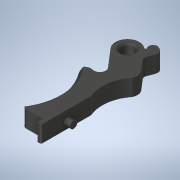
# Autodesk Inventor part: Trigger
Saved by Autodesk Inventor 2020.1 (Build 241239000, 239)
## iProperties
Created: 2019-07-16
Part Number: Trigger
Material: Generic
Document SubType Name: Modeling
Designer: Petar
Density: 1 g/cm^3
Appearance: Black Only
Mass: 1.77104 g
Surface Area: 13.1807 cm^2
Volume: 1.77104 cm^3
Author: Petar
Autodesk Inventor part; units mm, degrees
ref_plane "YZ Plane" through (0, 0, 0) normal (1, 0, 0) x (0, 1, 0)
ref_plane "XZ Plane" through (0, 0, 0) normal (0, 1, 0) x (-1, 0, 0)
sketch "Sketch1" plane through (0, 0, 0) normal (0, 1, 0) x (-1, 0, 0)
  arc A0 (0.6231, 32.7963) -> (2.0842, 14.5566) centre (15.636, 24.8205) ccw
  line L0 (-0.7016, 35) -> (-5.7016, 35)
  arc A1 (0.6231, 32.7963) -> (-0.7016, 35) centre (-0.7016, 33.5) ccw
  arc A2 (1.4227, 12.2493) -> (2.0842, 14.5566) centre (0.8884, 13.6509) ccw
  arc A3 (-9.0865, 8.0552) -> (-7.7016, 20) centre (-18.71, 15.2236) ccw
  line L1 (-7.7016, 37) -> (-7.7016, 20)
  arc A4 (-2.5532, -3.0792) -> (3.0381, 2.6019) centre (0, 0) ccw
  circle A5 centre (0, 0) radius 2.2
  arc A6 (-0.4832, 12.1334) -> (-2.3197, 8.8578) centre (-0.8007, 10.1588) ccw
  line L2 (3.0381, 2.6019) -> (-2.3197, 8.8578)
  line L3 (-5.8467, 0.6774) -> (-8.9592, 4.3116)
  arc A7 (-9.0865, 8.0552) -> (-8.9592, 4.3116) centre (-6.6806, 6.263) ccw
  line L4 (0, 0) -> (0, -31) construction
  line L5 (1.4227, 12.2493) -> (0.7686, 12)
  line L6 (-0.4832, 12.1334) -> (0.5112, 11.9735)
  arc A8 (0.5112, 11.9735) -> (0.7686, 12) centre (0.5905, 12.4672) ccw
  line L7 (3.7362, -42.8746) -> (-104.2638, 7.1254) construction
  line L8 (-104.2638, 7.1254) -> (-40.257, 145.38) construction
  line L9 (-40.257, 145.38) -> (67.743, 95.38) construction
  line L10 (67.743, 95.38) -> (3.7362, -42.8746) construction
  line L11 (-3.3359, -3.2768) -> (-4.3901, -5.8859) construction
  line L12 (-4.3901, -5.8859) -> (-7.1716, -4.7621)
  line L13 (-7.1716, -4.7621) -> (-5.5952, -0.8602)
  arc A9 (-5.5952, -0.8602) -> (-5.8467, 0.6774) centre (-6.986, -0.2983) ccw
  arc A10 (-2.5532, -3.0792) -> (-3.3359, -3.2768) centre (-2.8723, -3.4641) ccw
  line L14 (-7.7016, 37) -> (-6.2016, 37)
  line L15 (-6.2016, 37) -> (-6.2016, 35.5)
  arc A11 (-6.2016, 35.5) -> (-5.7016, 35) centre (-5.7016, 35.5) ccw
  arc A12 (-4.3901, -5.8859) -> (-3.3359, -3.2768) centre (-4.345, -4.3866) ccw
  point P0 (-7.7016, 35)
  point P1 (-3.0552, -2.5819)
  point P2 (-6.2016, 35)
  dimension "d5" = 7
  dimension "d6" = 15
  dimension "d7" = 8
  dimension "d8" = 4.4
  dimension "d9" = 2
  dimension "d10" = 35
  dimension "d14" = 3
  dimension "d18" = 12
  dimension "d93" = 3
  dimension "d94" = 1.5
  dimension "d96" = 22
  dimension "d109" = 0.5
  dimension "d115" = 0.7
  dimension "d116" = 150
  dimension "d121" = 0.5
  dimension "d123" = 1.5
  dimension "d124" = 2
  dimension "d140" = 1.5
  constraints: 25 point on circle, 24 end point, 18 tangent, 13 centre point, 5 point on line, 4 perpendicular, 3 coincident, 1 parallel, 1 vertical, 9 other
  measures "d5" distance of L0.start point (-7.702, 35)
  measures "d6" distance of point (-7.702, 35) L1.end
  measures "d7" diameter of A4
  measures "d8" diameter of A5
  measures "d9" radius of A6
  measures "d10" distance from line of L0 A4.centre
  measures "d14" radius of A7
  measures "d18" radius of A3
  measures "d93" distance between parallel lines of L13 L11
  measures "d94" radius of A9
  measures "d96" angle of L4 L11
  measures "d109" radius of A10
  measures "d115" distance of L5.start L5.end
  measures "d116" angle of L6 L5
  measures "d121" radius of A11
  measures "d123" distance of L1.start L14.end
  measures "d124" distance between parallel lines of L14 L0
  measures "d140" radius of A12
extrude "Extrusion1" add sketch "Sketch1" along normal mid plane 5.6
ref_plane "Work Plane1" through (-15.636, 0, 24.8205) normal (0, 0, -1) x (0, 1, 0)
sketch "Sketch2" plane through (-15.636, 0, 24.8205) normal (0, 0, -1) x (0, 1, 0)
  line L0 (-25.04, 0) -> (8.14, 0) construction
  line L1 (0, 15.636) -> (0, 0) construction
  line L2 (-19.6, 0) -> (3.3, 18.4018)
  line L3 (3.3, 18.4018) -> (3.3, 0)
  line L4 (2.8, 17) -> (2.8, 15.0129) construction
  line L5 (2.8, 17) -> (2.8, 18)
  line L6 (-2.8, 21.3376) -> (-2.8, 16.3376) construction
  line L7 (0, 15.75) -> (2.8, 15.75) construction
  point P0 (2.8, 13.5518)
  point P1 (-3, 20.3376)
  dimension "d101" = 1
  dimension "d103" = 0.5
  dimension "d110" = 1.25
  constraints: 10 end point, 5 point on line, 2 vertical, 1 horizontal, 1 perpendicular, 1 other
  measures "d101" distance of L4.start L5.end
  measures "d103" distance between parallel lines of L3 L4
  measures "d110" distance from line of L4.start L7
revolve "Revolution1" cut sketch "Sketch2" angle 360 about axis through (-15.636, 0, 24.8205) along (0, 1, 0) fills toward (-8.1187, 9.1619) open curves L2 L3
mirror "Mirror1" about plane through (0, 0, 0) normal (0, 1, 0) of "Revolution1"
chamfer "Chamfer1" distance 0.5 angle 45 2 edges at (2.2, 2.8, 0) (2.2, -2.8, 0)
sketch "Sketch4" plane through (0, -2.8, 0) normal (0, -1, 0) x (1, 0, 0)
  circle A0 centre (0, 0) radius 2.7 projected
  arc A1 (-3.0381, 2.6019) -> (2.5532, -3.0792) centre (0, 0) ccw projected
  arc A2 (2.5532, -3.0792) -> (-3.0381, 2.6019) centre (0, 0) ccw
  constraints: 2 point on circle, 1 centre point, 1 coincident
extrude "Extrusion3" add sketch "Sketch4" along normal blind 0.2
fillet "Fillet1" radius 0.5 2 edges at (6.2016, 0, 37) (7.7016, 0, 37)
fillet "Fillet2" radius 2 1 edges at (7.1716, 0, -4.7621)
sketch "Sketch3" plane through (7.7016, 0.2, 20) normal (1, 0, 0) x (0, 1, 0)
  circle A0 centre (-0.85, 8) radius 1.2
  line L0 (-3, 0) -> (2.6, 0) construction
  point P0 (-0.2, -20)
  dimension "d149" = 2.4
  dimension "d151" = 8
  dimension "d154" = 2.15
  constraints: 1 centre point
  measures "d149" diameter of A0
  measures "d151" distance from line of L0 A0.centre
  measures "d154" horizontal distance of L0.start A0.centre
extrude "Extrusion2" add sketch "Sketch3" along normal blind 2
body "Solid1"
